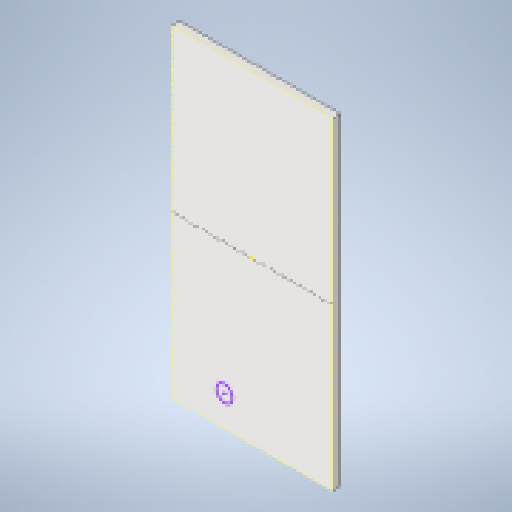
# Autodesk Inventor part: NDM 7.45 bracket middle plate 1
Saved by Autodesk Inventor 2025 (Build 290162010, 162A)
## iProperties
Created: 2023-07-04
Part Number: NDM 7.45 bracket middle plate 1
Material: Stainless Steel
Description: 2mm
Document SubType Name: Sheet Metal
Designer: DELL
Stock Number: NDM 7.1 папа ноги домкрат
Mass: 592.546 g
Surface Area: 766.755 cm^2
Volume: 74.0682 cm^3
Density: 8 g/cm^3
Flat Pattern Width: 3.5 cm
Flat Pattern Length: 8.5 cm
Flat Pattern Area: 29.75 cm^2
Sheet Metal Rule: Default_mm
Sheet Metal Width: 35,000 mm
Sheet Metal Length: 85,000 mm
Sheet Metal Area: 2975,000 mm^2
Appearance: Default
Author: user
Revision Number: 8
Autodesk Inventor part; units mm, degrees
ref_plane "YZ Plane" through (0, 0, 0) normal (1, 0, 0) x (0, 1, 0)
ref_plane "XZ Plane" through (0, 0, 0) normal (0, 1, 0) x (-1, 0, 0)
ref_plane "XY Plane" through (0, 0, 0) normal (0, 0, 1) x (1, 0, 0)
sketch "Sketch1" plane through (0, 0, 0) normal (0, 0, 1) x (1, 0, 0)
  line L0 (-17.5, 42.5) -> (17.5, 42.5)
  line L1 (17.5, 42.5) -> (17.5, -42.5)
  line L2 (17.5, -42.5) -> (-17.5, -42.5)
  line L3 (-17.5, -42.5) -> (-17.5, 42.5)
  line L4 (-17.5, 42.5) -> (17.5, -42.5) construction
  line L5 (17.5, 42.5) -> (-17.5, -42.5) construction
  point P0 (0, 0)
  point P1 (0, 0)
  dimension "d0" = 35
  dimension "d1" = 85
  constraints: 12 end point, 2 midpoint, 1 coincident, 1 horizontal, 1 parallel, 1 perpendicular
  measures "d0" distance of L1.end L2.end
  measures "d1" distance of L2.end L0.start
extrude "Plate1" add sketch "Sketch1" along normal blind 2
sketch "Sketch6" plane through (0, 0, 2) normal (0, 0, 1) x (1, 0, 0)
  line L0 (17.5, 42.5) -> (17.5, -42.5) projected
  line L1 (-17.5, 42.5) -> (17.5, 42.5) projected
  line L2 (-17.5, -42.5) -> (-17.5, 42.5) projected
  line L3 (17.5, -42.5) -> (-17.5, -42.5) projected
  circle A0 centre (0, -35) radius 3
  line L4 (-17.5, 0) -> (17.5, 0) construction
  line L5 (17.5, 42.5) -> (17.5, -42.5) projected
  circle A1 centre (0, 35) radius 3
  line L6 (7.5, -42.5) -> (17.5, -20)
  line L7 (-7.5, -42.5) -> (-17.5, -20)
  line L8 (-17.5, 20) -> (-7.5, 42.5)
  line L9 (17.5, 20) -> (7.5, 42.5)
  point P0 (0, 0)
  point P1 (0, 0)
  dimension "d36" = 70
  dimension "d37" = 6
  dimension "d43" = 40
  dimension "d44" = 15
  constraints: 10 end point, 8 point on line, 3 equal length, 3 midpoint, 2 centre point, 2 horizontal alignment, 1 vertical alignment, 2 other
  measures "d36" distance of A0.centre A1.centre
  measures "d37" diameter of A0
  measures "d43" distance of L8.start L7.end
  measures "d44" distance of L6.start L7.start
extrude "Cut1" cut sketch "Sketch6" against normal blind 2 contours L0 L9 L1 | L0 L3 L6 | L8 L2 L1 | L3 L2 L7 | A0 | A1
equation "\"d38\" = Thickness"
equation "\"d2\" = Thickness"
equation "\"BendRadius\" = Thickness"
equation "\"BendReliefWidth\" = Thickness"
equation "\"BendReliefDepth\" = 0.5 * Thickness"
equation "\"CornerReliefSize\" = 4 * Thickness"
equation "\"MinimumRemnant\" = 2 * Thickness"
equation "\"TransitionRadius\" = BendRadius"
equation "\"JacobiRadiusSize\" = BendRadius"
equation "\"GapSize\" = Thickness"
equation "\"Thickness\" = 2"
body "Solid1"
